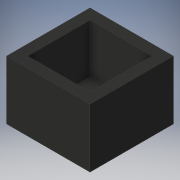
# Autodesk Inventor part: bar_protector
Saved by Autodesk Inventor 2019 (Build 230136000, 136)
## iProperties
Created: 2019-02-16
Part Number: bar_protector
Material: Rubber, Butyl
Document SubType Name: Modeling
Designer: suchanek
Density: 0.12 g/cm^3
Appearance: Rubber - Black
Author: suchanek
Autodesk Inventor part; units mm, degrees
ref_plane "YZ Plane" through (0, 0, 0) normal (1, 0, 0) x (0, 1, 0)
ref_plane "XZ Plane" through (0, 0, 0) normal (0, 1, 0) x (-1, 0, 0)
ref_plane "XY Plane" through (0, 0, 0) normal (0, 0, 1) x (1, 0, 0)
sketch "Sketch1" plane through (0, 0, 0) normal (0, 1, 0) x (-1, 0, 0)
  line L0 (-8.5, 8.5) -> (8.5, 8.5)
  line L1 (8.5, 8.5) -> (8.5, -8.5)
  line L2 (8.5, -8.5) -> (-8.5, -8.5)
  line L3 (-8.5, -8.5) -> (-8.5, 8.5)
  line L4 (-8.5, 8.5) -> (8.5, -8.5) construction
  line L5 (8.5, 8.5) -> (-8.5, -8.5) construction
  point P0 (0, 0)
  dimension "d0" = 17
  dimension "d1" = 17
  constraints: 12 end point, 2 midpoint, 2 parallel, 1 horizontal, 1 perpendicular
  measures "d0" distance of L1.end L2.end
  measures "d1" distance of L0.end L1.end
extrude "Extrusion1" add sketch "Sketch1" along normal blind 2
sketch "Sketch2" plane through (0, 2, 0) normal (0, 1, 0) x (1, 0, 0)
  line L0 (8.5, 8.5) -> (-8.5, 8.5) projected
  line L1 (8.5, -8.5) -> (-8.5, -8.5)
  line L2 (-8.5, -8.5) -> (-8.5, 8.5)
  line L3 (-8.5, 8.5) -> (8.5, 8.5)
  line L4 (8.5, 8.5) -> (8.5, -8.5)
  line L5 (8.5, -8.5) -> (-8.5, 8.5) construction
  line L6 (-8.5, -8.5) -> (8.5, 8.5) construction
  line L7 (6.35, -6.35) -> (-6.35, -6.35)
  line L8 (-6.35, -6.35) -> (-6.35, 6.35)
  line L9 (-6.35, 6.35) -> (6.35, 6.35)
  line L10 (6.35, 6.35) -> (6.35, -6.35)
  line L11 (6.35, -6.35) -> (-6.35, 6.35) construction
  line L12 (-6.35, -6.35) -> (6.35, 6.35) construction
  point P0 (0, 0)
  dimension "d4" = 12.7
  constraints: 24 end point, 4 midpoint, 4 parallel, 2 horizontal, 2 perpendicular, 1 point on line
  measures "d4" distance of L8.end L9.end
extrude "Extrusion2" add sketch "Sketch2" along normal blind 10
body "Solid1"
